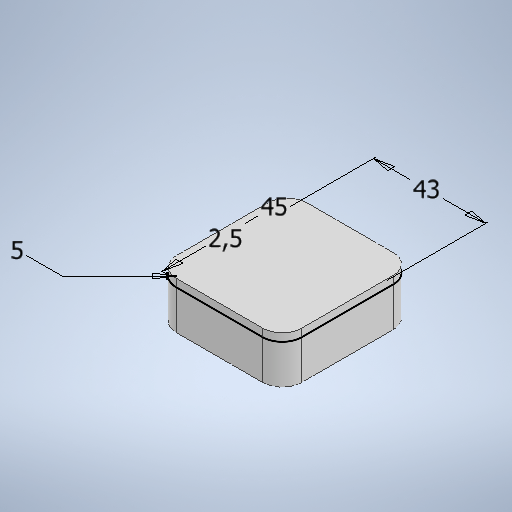
# Autodesk Inventor part: PCB_Deckel
Saved by Autodesk Inventor 2025.2 (Build 292293000, 293)
## iProperties
Created: 2024-11-12
Part Number: PCB_Deckel
Material: Generic
Document SubType Name: Modeling
Designer: matss
Density: 1 g/cm^3
Appearance: Default
Author: matss
Autodesk Inventor part; units mm, degrees
ref_plane "YZ Plane" through (0, 0, 0) normal (1, 0, 0) x (0, 1, 0)
ref_plane "XZ Plane" through (0, 0, 0) normal (0, 1, 0) x (-1, 0, 0)
ref_plane "XY Plane" through (0, 0, 0) normal (0, 0, 1) x (1, 0, 0)
sketch "Sketch1" plane through (0, 0, 0) normal (0, 1, 0) x (-1, 0, 0)
  line L0 (16.5, 22.5) -> (-16.5, 22.5)
  line L1 (-21.5, 17.5) -> (-21.5, -17.5)
  line L2 (-16.5, -22.5) -> (16.5, -22.5)
  line L3 (21.5, -17.5) -> (21.5, 17.5)
  arc A0 (21.5, 17.5) -> (16.5, 22.5) centre (16.5, 17.5) ccw
  arc A1 (16.5, -22.5) -> (21.5, -17.5) centre (16.5, -17.5) ccw
  arc A2 (-21.5, -17.5) -> (-16.5, -22.5) centre (-16.5, -17.5) ccw
  arc A3 (-16.5, 22.5) -> (-21.5, 17.5) centre (-16.5, 17.5) ccw
  line L4 (24, 17.5) -> (24, -17.5)
  arc A4 (16.5, -25) -> (24, -17.5) centre (16.5, -17.5) ccw
  line L5 (16.5, -25) -> (-16.5, -25)
  arc A5 (-24, -17.5) -> (-16.5, -25) centre (-16.5, -17.5) ccw
  line L6 (-24, -17.5) -> (-24, 17.5)
  arc A6 (-16.5, 25) -> (-24, 17.5) centre (-16.5, 17.5) ccw
  line L7 (-16.5, 25) -> (16.5, 25)
  arc A7 (24, 17.5) -> (16.5, 25) centre (16.5, 17.5) ccw
  point P0 (0, 0)
  point P1 (21.5, 22.5)
  point P2 (21.5, -22.5)
  point P3 (0, 22.5)
  point P4 (21.5, 0)
  dimension "d0" = 45
  dimension "d1" = 43
  dimension "d2" = 5
  dimension "d3" = 2.5
  constraints: 16 end point, 16 point on circle, 8 centre point, 8 tangent, 4 parallel, 4 point on line, 3 equal radius, 2 midpoint, 2 perpendicular, 1 horizontal, 1 horizontal alignment, 1 vertical alignment, 7 other
  measures "d0" distance of point (21.5, -22.5) point (21.5, 22.5)
  measures "d1" distance between parallel lines of L1 L3
  measures "d2" radius of A0
  measures "d3" distance between parallel lines of L3 L4
extrude "Extrusion1" add sketch "Sketch1" along normal blind 3 contours A0 L3 A1 L2 A2 L1 A3 L0 | L4 A4 L5 A5 L6 A6 L7 A7
extrude "Extrusion2" add sketch "Sketch1" against normal blind 15
body "Solid1"
